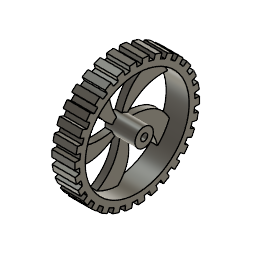
wheel (Autodesk Fusion 360 design; units mm, degrees)
part number: 2026-01-28-15-37-27-718
Autodesk Fusion 360 part; units mm, degrees
sketch "Sketch1" plane through (0, 0, 0) normal (1, 0, 0) x (0, 1, 0)
  circle A0 centre (0, 0) radius 25
  circle A1 centre (0, 0) radius 22.5
  line L0 (-24.9947, -0.514) -> (-26.9947, -0.514)
  line L1 (-26.9947, -0.514) -> (-26.9947, 2.5)
  line L2 (-26.9947, 2.5) -> (-24.8747, 2.5)
  line L3 (-26.2979, -6.1153) -> (-26.9246, -3.1671)
  line L4 (-26.9246, -3.1671) -> (-24.8509, -2.7264)
  line L5 (-24.3416, -5.6995) -> (-26.2979, -6.1153)
  line L6 (-24.4518, -11.4493) -> (-25.6777, -8.6959)
  line L7 (-25.6777, -8.6959) -> (-23.741, -7.8336)
  line L8 (-22.6247, -10.6359) -> (-24.4518, -11.4493)
  line L9 (-21.537, -16.283) -> (-23.3086, -13.8446)
  line L10 (-23.3086, -13.8446) -> (-21.5935, -12.5984)
  line L11 (-19.919, -15.1074) -> (-21.537, -16.283)
  line L12 (-17.681, -20.4049) -> (-19.9209, -18.3882)
  line L13 (-19.9209, -18.3882) -> (-18.5023, -16.8127)
  line L14 (-16.3427, -18.9186) -> (-17.681, -20.4049)
  line L15 (-13.0522, -23.6351) -> (-15.6624, -22.1281)
  line L16 (-15.6624, -22.1281) -> (-14.6024, -20.2921)
  line L17 (-12.0522, -21.9031) -> (-13.0522, -23.6351)
  line L18 (-7.853, -25.8323) -> (-10.7195, -24.901)
  line L19 (-10.7195, -24.901) -> (-10.0643, -22.8847)
  line L20 (-7.2349, -23.9302) -> (-7.853, -25.8323)
  line L21 (-2.3105, -26.9006) -> (-5.308, -26.5855)
  line L22 (-5.308, -26.5855) -> (-5.0864, -24.4771)
  line L23 (-2.1014, -24.9115) -> (-2.3105, -26.9006)
  line L24 (3.3329, -26.7931) -> (0.3354, -27.1082)
  line L25 (0.3354, -27.1082) -> (0.1138, -24.9997)
  line L26 (3.1239, -24.8041) -> (3.3329, -26.7931)
  line L27 (8.8307, -25.5147) -> (5.9642, -26.446)
  line L28 (5.9642, -26.446) -> (5.3091, -24.4298)
  line L29 (8.2127, -23.6125) -> (8.8307, -25.5147)
  line L30 (13.9425, -23.1211) -> (11.3323, -24.6281)
  line L31 (11.3323, -24.6281) -> (10.2723, -22.7921)
  line L32 (12.9425, -21.389) -> (13.9425, -23.1211)
  line L33 (18.445, -19.717) -> (16.2051, -21.7338)
  line L34 (16.2051, -21.7338) -> (14.7866, -20.1583)
  line L35 (17.1067, -18.2307) -> (18.445, -19.717)
  line L36 (22.1413, -15.4512) -> (20.3697, -17.8896)
  line L37 (20.3697, -17.8896) -> (18.6546, -16.6435)
  line L38 (20.5233, -14.2757) -> (22.1413, -15.4512)
  line L39 (24.87, -10.5102) -> (23.6441, -13.2636)
  line L40 (23.6441, -13.2636) -> (21.7073, -12.4013)
  line L41 (23.0429, -9.6967) -> (24.87, -10.5102)
  line L42 (26.5117, -5.1097) -> (25.885, -8.0579)
  line L43 (25.885, -8.0579) -> (23.8113, -7.6171)
  line L44 (24.5554, -4.6939) -> (26.5117, -5.1097)
  line L45 (26.9947, 0.514) -> (26.9947, -2.5)
  line L46 (26.9947, -2.5) -> (24.8747, -2.5)
  line L47 (24.9947, 0.514) -> (26.9947, 0.514)
  line L48 (26.2979, 6.1153) -> (26.9246, 3.1671)
  line L49 (26.9246, 3.1671) -> (24.8509, 2.7264)
  line L50 (24.3416, 5.6995) -> (26.2979, 6.1153)
  line L51 (24.4518, 11.4493) -> (25.6777, 8.6959)
  line L52 (25.6777, 8.6959) -> (23.741, 7.8336)
  line L53 (22.6247, 10.6359) -> (24.4518, 11.4493)
  line L54 (21.537, 16.283) -> (23.3086, 13.8446)
  line L55 (23.3086, 13.8446) -> (21.5935, 12.5984)
  line L56 (19.919, 15.1074) -> (21.537, 16.283)
  line L57 (17.681, 20.4049) -> (19.9209, 18.3882)
  line L58 (19.9209, 18.3882) -> (18.5023, 16.8127)
  line L59 (16.3427, 18.9186) -> (17.681, 20.4049)
  line L60 (13.0522, 23.6351) -> (15.6624, 22.1281)
  line L61 (15.6624, 22.1281) -> (14.6024, 20.2921)
  line L62 (12.0522, 21.9031) -> (13.0522, 23.6351)
  line L63 (7.853, 25.8323) -> (10.7195, 24.901)
  line L64 (10.7195, 24.901) -> (10.0643, 22.8847)
  line L65 (7.2349, 23.9302) -> (7.853, 25.8323)
  line L66 (2.3105, 26.9006) -> (5.308, 26.5855)
  line L67 (5.308, 26.5855) -> (5.0864, 24.4771)
  line L68 (2.1014, 24.9115) -> (2.3105, 26.9006)
  line L69 (-3.3329, 26.7931) -> (-0.3354, 27.1082)
  line L70 (-0.3354, 27.1082) -> (-0.1138, 24.9997)
  line L71 (-3.1239, 24.8041) -> (-3.3329, 26.7931)
  line L72 (-8.8307, 25.5147) -> (-5.9642, 26.446)
  line L73 (-5.9642, 26.446) -> (-5.3091, 24.4298)
  line L74 (-8.2127, 23.6125) -> (-8.8307, 25.5147)
  line L75 (-13.9425, 23.1211) -> (-11.3323, 24.6281)
  line L76 (-11.3323, 24.6281) -> (-10.2723, 22.7921)
  line L77 (-12.9425, 21.389) -> (-13.9425, 23.1211)
  line L78 (-18.445, 19.717) -> (-16.2051, 21.7338)
  line L79 (-16.2051, 21.7338) -> (-14.7866, 20.1583)
  line L80 (-17.1067, 18.2307) -> (-18.445, 19.717)
  line L81 (-22.1413, 15.4512) -> (-20.3697, 17.8896)
  line L82 (-20.3697, 17.8896) -> (-18.6546, 16.6435)
  line L83 (-20.5233, 14.2757) -> (-22.1413, 15.4512)
  line L84 (-24.87, 10.5102) -> (-23.6441, 13.2636)
  line L85 (-23.6441, 13.2636) -> (-21.7073, 12.4013)
  line L86 (-23.0429, 9.6967) -> (-24.87, 10.5102)
  line L87 (-26.5117, 5.1097) -> (-25.885, 8.0579)
  line L88 (-25.885, 8.0579) -> (-23.8113, 7.6171)
  line L89 (-24.5554, 4.6939) -> (-26.5117, 5.1097)
  circle A2 centre (0, 0) radius 1.5
  circle A3 centre (0, 0) radius 4
  spline S0 degree 5 poles (-1.9492, 3.4929) (-2.1542, 3.8682) (-2.5487, 4.6186) (-3.0944, 5.7442) (-3.7283, 7.245) (-4.3537, 9.1209) (-4.7968, 10.9968) (-5.0424, 12.8726) (-5.0811, 14.7484) (-4.9198, 16.624) (-4.5732, 18.4996) (-4.1596, 20.0001) (-3.7775, 21.1254) (-3.4914, 21.8756) (-3.3405, 22.2506) knots 0 0 0 0 0 0 0.1 0.2 0.3 0.4 0.5 0.6 0.7 0.8 0.9 1 1 1 1 1 1
  spline S1 degree 5 poles (-3.6854, 1.5549) (-4.0719, 1.8523) (-4.8263, 2.4516) (-5.9017, 3.3636) (-7.2214, 4.6064) (-8.6676, 6.2076) (-9.8908, 7.8611) (-10.8705, 9.5716) (-11.5921, 11.3427) (-12.0601, 13.1733) (-12.2915, 15.0593) (-12.3018, 16.6091) (-12.2172, 17.7931) (-12.1205, 18.5919) (-12.062, 18.9936) knots 0 0 0 0 0 0 0.1 0.2 0.3 0.4 0.5 0.6 0.7 0.8 0.9 1 1 1 1 1 1
  spline S2 degree 5 poles (-3.9243, -0.7744) (-4.3445, -0.8534) (-5.1801, -0.9967) (-6.4193, -1.1679) (-8.0425, -1.307) (-10.0199, -1.3221) (-11.9409, -1.1639) (-13.8008, -0.8178) (-15.5967, -0.2749) (-17.3307, 0.4581) (-19.0074, 1.3673) (-20.3066, 2.2243) (-21.2587, 2.9354) (-21.8838, 3.4394) (-22.1939, 3.6988) knots 0 0 0 0 0 0 0.1 0.2 0.3 0.4 0.5 0.6 0.7 0.8 0.9 1 1 1 1 1 1
  spline S3 degree 5 poles (-2.6177, -3.0245) (-3.02, -3.3002) (-3.823, -3.8325) (-5.0227, -4.5734) (-6.6125, -5.4445) (-8.5822, -6.3251) (-10.5327, -6.9775) (-12.4623, -7.3807) (-14.3697, -7.5196) (-16.2553, -7.3991) (-18.1205, -7.0364) (-19.5977, -6.5672) (-20.6976, -6.1209) (-21.4274, -5.782) (-21.7914, -5.6023) knots 0 0 0 0 0 0 0.1 0.2 0.3 0.4 0.5 0.6 0.7 0.8 0.9 1 1 1 1 1 1
  spline S4 degree 5 poles (-0.4762, -3.9716) (-0.5309, -4.3956) (-0.6528, -5.2346) (-0.8729, -6.466) (-1.2422, -8.0528) (-1.839, -9.938) (-2.583, -11.7161) (-3.4869, -13.378) (-4.5582, -14.9183) (-5.7911, -16.3409) (-7.174, -17.6546) (-8.3905, -18.6253) (-9.3611, -19.3112) (-10.0335, -19.7499) (-10.3761, -19.9646) knots 0 0 0 0 0 0 0.1 0.2 0.3 0.4 0.5 0.6 0.7 0.8 0.9 1 1 1 1 1 1
  spline S5 degree 5 poles (2.0676, -3.4242) (2.2055, -3.892) (2.4635, -4.8202) (2.7975, -6.1901) (3.1347, -7.9713) (3.3635, -10.1167) (3.3812, -12.1734) (3.1684, -14.1332) (2.7111, -15.9901) (2.0138, -17.7462) (1.0924, -19.408) (0.1898, -20.6679) (-0.5746, -21.576) (-1.1224, -22.1654) (-1.4058, -22.456) knots 0 0 0 0 0 0 0.1 0.2 0.3 0.4 0.5 0.6 0.7 0.8 0.9 1 1 1 1 1 1
  spline S6 degree 5 poles (3.63, -1.6801) (4.0164, -1.8632) (4.7767, -2.2384) (5.8798, -2.8283) (7.2748, -3.6699) (8.8833, -4.82) (10.3445, -6.0771) (11.6457, -7.4503) (12.7795, -8.9451) (13.7516, -10.5573) (14.5736, -12.2784) (15.1209, -13.7354) (15.4733, -14.8704) (15.6827, -15.6455) (15.7811, -16.0377) knots 0 0 0 0 0 0 0.1 0.2 0.3 0.4 0.5 0.6 0.7 0.8 0.9 1 1 1 1 1 1
  spline S7 degree 5 poles (3.8955, 0.9083) (4.383, 0.8948) (5.3456, 0.8534) (6.7516, 0.7477) (8.5498, 0.518) (10.661, 0.0726) (12.6224, -0.5461) (14.4205, -1.3541) (16.0453, -2.3628) (17.4999, -3.5687) (18.7957, -4.9584) (19.7149, -6.2062) (20.3424, -7.2138) (20.7337, -7.9169) (20.9225, -8.2763) knots 0 0 0 0 0 0 0.1 0.2 0.3 0.4 0.5 0.6 0.7 0.8 0.9 1 1 1 1 1 1
  spline S8 degree 5 poles (2.7197, 2.9332) (3.0132, 3.244) (3.6049, 3.8512) (4.5068, 4.718) (5.7383, 5.7847) (7.3292, 6.9591) (8.9763, 7.9603) (10.6844, 8.7735) (12.4564, 9.3899) (14.2901, 9.8161) (16.181, 10.0661) (17.7358, 10.1364) (18.9241, 10.1207) (19.726, 10.0804) (20.1294, 10.0528) knots 0 0 0 0 0 0 0.1 0.2 0.3 0.4 0.5 0.6 0.7 0.8 0.9 1 1 1 1 1 1
  spline S9 degree 5 poles (0.34, 3.9855) (0.5034, 4.445) (0.8402, 5.3477) (1.3753, 6.6522) (2.1494, 8.2914) (3.2253, 10.1616) (4.4199, 11.8359) (5.744, 13.2963) (7.2054, 14.5298) (8.8017, 15.5406) (10.5239, 16.3435) (11.9947, 16.8322) (13.1469, 17.1176) (13.9365, 17.2724) (14.3367, 17.341) knots 0 0 0 0 0 0 0.1 0.2 0.3 0.4 0.5 0.6 0.7 0.8 0.9 1 1 1 1 1 1
  point P0 (-5, 13)
  point P1 (-11, 10)
  point P2 (-13.9088, -0.7381)
  point P3 (-12.9098, -7.3715)
  point P4 (-3.5961, -13.4561)
  point P5 (3.0213, -14.5558)
  point P6 (11.6863, -7.5783)
  point P7 (14.777, -1.6245)
  point P8 (10.8186, 8.7725)
  point P9 (6.1114, 13.5518)
  dimension "d1" = 50
  dimension "d2" = 45
  dimension "d3" = 2
  dimension "d5" = 360
  dimension "d6" = 3
  dimension "d7" = 8
  dimension "d9" = 360
  constraint coincident A0.centre A1.centre
  constraint coincident A0 L0.start
  constraint horizontal L0
  constraint perpendicular L0 L1
  constraint coincident A0 L2.end
  constraint perpendicular L1 L2
  constraint concentric A0 A2
  constraint concentric A0 A3
  constraint coincident A3 S0.start
  constraint coincident A1 S0.end
  constraint coincident A3 S1.start
  constraint coincident A1 S1.end
  measures "d1" diameter of A0
  measures "d2" diameter of A1
  measures "d3" distance of L0.start L0.end
  measures "d6" diameter of A2
  measures "d7" diameter of A3
extrude "Extrude1" add sketch "Sketch1" along normal blind 10 contours A0 | A0 L45 L46 L47 | A0 L48 L49 L50 | A0 L42 L43 L44 | A0 L51 L52 L53 | A0 L39 L40 L41 | A0 L54 L55 L56 | A0 L36 L37 L38 | A0 L57 L58 L59 | A0 L33 L34 L35 | A0 L60 L61 L62 | A0 L30 L31 L32 | A0 L63 L64 L65 | A0 L27 L28 L29 | A0 L66 L67 L68 | A0 L24 L25 L26 | A0 L69 L70 L71 | A0 L21 L22 L23 | A0 L72 L73 L74 | A0 L18 L19 L20 | A0 L75 L76 L77 | A0 L15 L16 L17 | A0 L78 L79 L80 | A0 L12 L13 L14 | A0 L81 L82 L83 | A0 L9 L10 L11 | A0 L84 L85 L86 | A0 L6 L7 L8 | A0 L87 L88 L89 | A0 L3 L4 L5 | A0 L0 L1 L2 makes body 1
extrude "Extrude2" add sketch "Sketch1" along normal blind 13 separate body contours A3 makes body 2
extrude "Extrude3" add sketch "Sketch1" against normal blind 1 separate body contours A2 makes body 3
extrude "Extrude4" add sketch "Sketch1" along normal blind 3 contours A1 A3 S8 S9 | A1 A3 S6 S7 | A1 A3 S0 S1 | A1 A3 S4 S5 | A1 A3 S2 S3 bodies 1 3 2
